Autodesk Fusion 360 part; units mm, degrees
note: some values were not read from the file. Set by a fixed rule: which sketch regions a step uses.
(part 3 of 3)
sketch "Sketch6" plane through (0, 0, 1) normal (0, 0, 1) x (-1, 0, 0)
  line L0 (-21.6697, -74.1094) -> (-35.669, -74.1094)
  line L1 (-35.669, -74.1094) -> (-35.669, -73.5101)
  line L2 (-35.669, -73.5101) -> (-36.4698, -73.5101)
  line L3 (-36.4698, -73.5101) -> (-36.4698, -60.7109)
  line L4 (-36.4698, -60.7109) -> (-35.669, -60.7109)
  line L5 (-35.669, -60.7109) -> (-35.669, -60.1102)
  line L6 (-35.669, -60.1102) -> (-21.6697, -60.1102)
  line L7 (-21.6697, -60.1102) -> (-21.6697, -60.7109)
  line L8 (-21.6697, -60.7109) -> (-20.869, -60.7109)
  line L9 (-20.869, -60.7109) -> (-20.869, -73.5101)
  line L10 (-20.869, -73.5101) -> (-21.6697, -73.5101)
  line L11 (-21.6697, -73.5101) -> (-21.6697, -74.1094)
  line L12 (-66.27, -35.585) -> (-69.07, -35.585)
  line L13 (-69.07, -35.585) -> (-69.07, -34.7597)
  line L14 (-69.07, -34.7597) -> (-72.3, -34.7597)
  line L15 (-72.3, -34.7597) -> (-72.3, -28.01)
  line L16 (-72.3, -28.01) -> (-69.07, -28.01)
  line L17 (-69.07, -28.01) -> (-69.07, -27.2852)
  line L18 (-69.07, -27.2852) -> (-73.1696, -27.2852)
  line L19 (-73.1696, -27.2852) -> (-73.1696, -26.4845)
  line L20 (-73.1696, -26.4845) -> (-73.769, -26.4845)
  line L21 (-73.769, -26.4845) -> (-73.769, -12.485)
  line L22 (-73.769, -12.485) -> (-73.1696, -12.485)
  line L23 (-73.1696, -12.485) -> (-73.1696, -11.6858)
  line L24 (-73.1696, -11.6858) -> (-69.07, -11.6858)
  line L25 (-69.07, -11.6858) -> (-69.07, -10.9595)
  line L26 (-69.07, -10.9595) -> (-72.3, -10.9595)
  line L27 (-72.3, -10.9595) -> (-72.3, -4.2099)
  line L28 (-72.3, -4.2099) -> (-69.07, -4.2099)
  line L29 (-69.07, -4.2099) -> (-69.07, -3.3858)
  line L30 (-69.07, -3.3858) -> (-66.27, -3.3858)
  line L31 (-66.27, -3.3858) -> (-66.27, -4.2099)
  line L32 (-66.27, -4.2099) -> (-59.9997, -4.2099)
  line L33 (-59.9997, -4.2099) -> (-59.9997, -5.9352)
  line L34 (-59.9997, -5.9352) -> (-58.7996, -5.9352)
  line L35 (-58.7996, -5.9352) -> (-58.7996, -9.2356)
  line L36 (-58.7996, -9.2356) -> (-59.9997, -9.2356)
  line L37 (-59.9997, -9.2356) -> (-59.9997, -10.9595)
  line L38 (-59.9997, -10.9595) -> (-64.4701, -10.9595)
  line L39 (-64.4701, -10.9595) -> (-64.4701, -11.6858)
  line L40 (-64.4701, -11.6858) -> (-60.3691, -11.6858)
  line L41 (-60.3691, -11.6858) -> (-60.3691, -12.485)
  line L42 (-60.3691, -12.485) -> (-59.7697, -12.485)
  line L43 (-59.7697, -12.485) -> (-59.7697, -26.4845)
  line L44 (-59.7697, -26.4845) -> (-60.3691, -26.4845)
  line L45 (-60.3691, -26.4845) -> (-60.3691, -27.2852)
  line L46 (-60.3691, -27.2852) -> (-64.4701, -27.2852)
  line L47 (-64.4701, -27.2852) -> (-64.4701, -28.01)
  line L48 (-64.4701, -28.01) -> (-59.9997, -28.01)
  line L49 (-59.9997, -28.01) -> (-59.9997, -29.7353)
  line L50 (-59.9997, -29.7353) -> (-58.7996, -29.7353)
  line L51 (-58.7996, -29.7353) -> (-58.7996, -33.0357)
  line L52 (-58.7996, -33.0357) -> (-59.9997, -33.0357)
  line L53 (-59.9997, -33.0357) -> (-59.9997, -34.7597)
  line L54 (-59.9997, -34.7597) -> (-66.27, -34.7597)
  line L55 (-66.27, -34.7597) -> (-66.27, -35.585)
  line L56 (-21.6697, -93.1594) -> (-35.669, -93.1594)
  line L57 (-35.669, -93.1594) -> (-35.669, -92.5601)
  line L58 (-35.669, -92.5601) -> (-36.4698, -92.5601)
  line L59 (-36.4698, -92.5601) -> (-36.4698, -79.7609)
  line L60 (-36.4698, -79.7609) -> (-35.669, -79.7609)
  line L61 (-35.669, -79.7609) -> (-35.669, -79.1602)
  line L62 (-35.669, -79.1602) -> (-21.6697, -79.1602)
  line L63 (-21.6697, -79.1602) -> (-21.6697, -79.7609)
  line L64 (-21.6697, -79.7609) -> (-20.869, -79.7609)
  line L65 (-20.869, -79.7609) -> (-20.869, -92.5601)
  line L66 (-20.869, -92.5601) -> (-21.6697, -92.5601)
  line L67 (-21.6697, -92.5601) -> (-21.6697, -93.1594)
  line L68 (-59.7697, -131.259) -> (-73.769, -131.259)
  line L69 (-73.769, -131.259) -> (-73.769, -130.66)
  line L70 (-73.769, -130.66) -> (-74.5698, -130.66)
  line L71 (-74.5698, -130.66) -> (-74.5698, -117.861)
  line L72 (-74.5698, -117.861) -> (-73.769, -117.861)
  line L73 (-73.769, -117.861) -> (-73.769, -117.26)
  line L74 (-73.769, -117.26) -> (-59.7697, -117.26)
  line L75 (-59.7697, -117.26) -> (-59.7697, -117.861)
  line L76 (-59.7697, -117.861) -> (-58.9689, -117.861)
  line L77 (-58.9689, -117.861) -> (-58.9689, -130.66)
  line L78 (-58.9689, -130.66) -> (-59.7697, -130.66)
  line L79 (-59.7697, -130.66) -> (-59.7697, -131.259)
  line L80 (-66.27, -73.685) -> (-69.07, -73.685)
  line L81 (-69.07, -73.685) -> (-69.07, -72.8595)
  line L82 (-69.07, -72.8595) -> (-72.3, -72.8595)
  line L83 (-72.3, -72.8595) -> (-72.3, -66.1098)
  line L84 (-72.3, -66.1098) -> (-69.07, -66.1098)
  line L85 (-69.07, -66.1098) -> (-69.07, -65.3852)
  line L86 (-69.07, -65.3852) -> (-73.1696, -65.3852)
  line L87 (-73.1696, -65.3852) -> (-73.1696, -64.5844)
  line L88 (-73.1696, -64.5844) -> (-73.769, -64.5844)
  line L89 (-73.769, -64.5844) -> (-73.769, -50.5852)
  line L90 (-73.769, -50.5852) -> (-73.1696, -50.5852)
  line L91 (-73.1696, -50.5852) -> (-73.1696, -49.7858)
  line L92 (-73.1696, -49.7858) -> (-69.07, -49.7858)
  line L93 (-69.07, -49.7858) -> (-69.07, -49.0594)
  line L94 (-69.07, -49.0594) -> (-72.3, -49.0594)
  line L95 (-72.3, -49.0594) -> (-72.3, -42.31)
  line L96 (-72.3, -42.31) -> (-69.07, -42.31)
  line L97 (-69.07, -42.31) -> (-69.07, -41.486)
  line L98 (-69.07, -41.486) -> (-66.27, -41.486)
  line L99 (-66.27, -41.486) -> (-66.27, -42.31)
  line L100 (-66.27, -42.31) -> (-59.9997, -42.31)
  line L101 (-59.9997, -42.31) -> (-59.9997, -44.0351)
  line L102 (-59.9997, -44.0351) -> (-58.7996, -44.0351)
  line L103 (-58.7996, -44.0351) -> (-58.7996, -47.3357)
  line L104 (-58.7996, -47.3357) -> (-59.9997, -47.3357)
  line L105 (-59.9997, -47.3357) -> (-59.9997, -49.0594)
  line L106 (-59.9997, -49.0594) -> (-64.4701, -49.0594)
  line L107 (-64.4701, -49.0594) -> (-64.4701, -49.7858)
  line L108 (-64.4701, -49.7858) -> (-60.3691, -49.7858)
  line L109 (-60.3691, -49.7858) -> (-60.3691, -50.5852)
  line L110 (-60.3691, -50.5852) -> (-59.7697, -50.5852)
  line L111 (-59.7697, -50.5852) -> (-59.7697, -64.5844)
  line L112 (-59.7697, -64.5844) -> (-60.3691, -64.5844)
  line L113 (-60.3691, -64.5844) -> (-60.3691, -65.3852)
  line L114 (-60.3691, -65.3852) -> (-64.4701, -65.3852)
  line L115 (-64.4701, -65.3852) -> (-64.4701, -66.1098)
  line L116 (-64.4701, -66.1098) -> (-59.9997, -66.1098)
  line L117 (-59.9997, -66.1098) -> (-59.9997, -67.8353)
  line L118 (-59.9997, -67.8353) -> (-58.7996, -67.8353)
  line L119 (-58.7996, -67.8353) -> (-58.7996, -71.1359)
  line L120 (-58.7996, -71.1359) -> (-59.9997, -71.1359)
  line L121 (-59.9997, -71.1359) -> (-59.9997, -72.8595)
  line L122 (-59.9997, -72.8595) -> (-66.27, -72.8595)
  line L123 (-66.27, -72.8595) -> (-66.27, -73.685)
  line L124 (-2.6197, -74.1094) -> (-16.6192, -74.1094)
  line L125 (-16.6192, -74.1094) -> (-16.6192, -73.5101)
  line L126 (-16.6192, -73.5101) -> (-17.4198, -73.5101)
  line L127 (-17.4198, -73.5101) -> (-17.4198, -60.7109)
  line L128 (-17.4198, -60.7109) -> (-16.6192, -60.7109)
  line L129 (-16.6192, -60.7109) -> (-16.6192, -60.1102)
  line L130 (-16.6192, -60.1102) -> (-2.6196, -60.1102)
  line L131 (-2.6197, -60.1102) -> (-2.6197, -60.7109)
  line L132 (-2.6197, -60.7109) -> (-1.819, -60.7109)
  line L133 (-1.819, -60.7109) -> (-1.819, -73.5101)
  line L134 (-1.819, -73.5101) -> (-2.6197, -73.5101)
  line L135 (-2.6197, -73.5101) -> (-2.6197, -74.1094)
  line L136 (-59.7697, -93.1594) -> (-73.769, -93.1594)
  line L137 (-73.769, -93.1594) -> (-73.769, -92.5601)
  line L138 (-73.769, -92.5601) -> (-74.5698, -92.5601)
  line L139 (-74.5698, -92.5601) -> (-74.5698, -79.7609)
  line L140 (-74.5698, -79.7609) -> (-73.769, -79.7609)
  line L141 (-73.769, -79.7609) -> (-73.769, -79.1602)
  line L142 (-73.769, -79.1602) -> (-59.7697, -79.1602)
  line L143 (-59.7697, -79.1602) -> (-59.7697, -79.7609)
  line L144 (-59.7697, -79.7609) -> (-58.9689, -79.7609)
  line L145 (-58.9689, -79.7609) -> (-58.9689, -92.5601)
  line L146 (-58.9689, -92.5601) -> (-59.7697, -92.5601)
  line L147 (-59.7697, -92.5601) -> (-59.7697, -93.1594)
  line L148 (-40.7197, -93.1594) -> (-54.719, -93.1594)
  line L149 (-54.719, -93.1594) -> (-54.719, -92.5601)
  line L150 (-54.719, -92.5601) -> (-55.5198, -92.5601)
  line L151 (-55.5198, -92.5601) -> (-55.5198, -79.7609)
  line L152 (-55.5198, -79.7609) -> (-54.719, -79.7609)
  line L153 (-54.719, -79.7609) -> (-54.719, -79.1602)
  line L154 (-54.719, -79.1602) -> (-40.7197, -79.1602)
  line L155 (-40.7197, -79.1602) -> (-40.7197, -79.7609)
  line L156 (-40.7197, -79.7609) -> (-39.9189, -79.7609)
  line L157 (-39.9189, -79.7609) -> (-39.9189, -92.5601)
  line L158 (-39.9189, -92.5601) -> (-40.7197, -92.5601)
  line L159 (-40.7197, -92.5601) -> (-40.7197, -93.1594)
  line L160 (-2.6197, -36.0094) -> (-16.6192, -36.0094)
  line L161 (-16.6192, -36.0094) -> (-16.6192, -35.4101)
  line L162 (-16.6192, -35.4101) -> (-17.4198, -35.4101)
  line L163 (-17.4198, -35.4101) -> (-17.4198, -22.6109)
  line L164 (-17.4198, -22.6109) -> (-16.6192, -22.6109)
  line L165 (-16.6192, -22.6109) -> (-16.6192, -22.01)
  line L166 (-16.6192, -22.01) -> (-2.6196, -22.01)
  line L167 (-2.6197, -22.01) -> (-2.6197, -22.6109)
  line L168 (-2.6197, -22.6109) -> (-1.819, -22.6109)
  line L169 (-1.819, -22.6109) -> (-1.819, -35.4101)
  line L170 (-1.819, -35.4101) -> (-2.6197, -35.4101)
  line L171 (-2.6197, -35.4101) -> (-2.6197, -36.0094)
  line L172 (-2.6197, -55.0594) -> (-16.6192, -55.0594)
  line L173 (-16.6192, -55.0594) -> (-16.6192, -54.4601)
  line L174 (-16.6192, -54.4601) -> (-17.4198, -54.4601)
  line L175 (-17.4198, -54.4601) -> (-17.4198, -41.6609)
  line L176 (-17.4198, -41.6609) -> (-16.6192, -41.6609)
  line L177 (-16.6192, -41.6609) -> (-16.6192, -41.0602)
  line L178 (-16.6192, -41.0602) -> (-2.6196, -41.0602)
  line L179 (-2.6197, -41.0602) -> (-2.6197, -41.6609)
  line L180 (-2.6197, -41.6609) -> (-1.819, -41.6609)
  line L181 (-1.819, -41.6609) -> (-1.819, -54.4601)
  line L182 (-1.819, -54.4601) -> (-2.6197, -54.4601)
  line L183 (-2.6197, -54.4601) -> (-2.6197, -55.0594)
  line L184 (-21.6697, -55.0594) -> (-35.669, -55.0594)
  line L185 (-35.669, -55.0594) -> (-35.669, -54.4601)
  line L186 (-35.669, -54.4601) -> (-36.4698, -54.4601)
  line L187 (-36.4698, -54.4601) -> (-36.4698, -41.6609)
  line L188 (-36.4698, -41.6609) -> (-35.669, -41.6609)
  line L189 (-35.669, -41.6609) -> (-35.669, -41.0602)
  line L190 (-35.669, -41.0602) -> (-21.6697, -41.0602)
  line L191 (-21.6697, -41.0602) -> (-21.6697, -41.6609)
  line L192 (-21.6697, -41.6609) -> (-20.869, -41.6609)
  line L193 (-20.869, -41.6609) -> (-20.869, -54.4601)
  line L194 (-20.869, -54.4601) -> (-21.6697, -54.4601)
  line L195 (-21.6697, -54.4601) -> (-21.6697, -55.0594)
  line L196 (-40.7197, -74.1094) -> (-54.719, -74.1094)
  line L197 (-54.719, -74.1094) -> (-54.719, -73.5101)
  line L198 (-54.719, -73.5101) -> (-55.5198, -73.5101)
  line L199 (-55.5198, -73.5101) -> (-55.5198, -60.7109)
  line L200 (-55.5198, -60.7109) -> (-54.719, -60.7109)
  line L201 (-54.719, -60.7109) -> (-54.719, -60.1102)
  line L202 (-54.719, -60.1102) -> (-40.7197, -60.1102)
  line L203 (-40.7197, -60.1102) -> (-40.7197, -60.7109)
  line L204 (-40.7197, -60.7109) -> (-39.9189, -60.7109)
  line L205 (-39.9189, -60.7109) -> (-39.9189, -73.5101)
  line L206 (-39.9189, -73.5101) -> (-40.7197, -73.5101)
  line L207 (-40.7197, -73.5101) -> (-40.7197, -74.1094)
  line L208 (-12.1447, -16.9595) -> (-26.1441, -16.9595)
  line L209 (-26.1441, -16.9595) -> (-26.1441, -16.3601)
  line L210 (-26.1441, -16.3601) -> (-26.9448, -16.3601)
  line L211 (-26.9448, -16.3601) -> (-26.9448, -12.2604)
  line L212 (-26.9448, -12.2604) -> (-27.6696, -12.2604)
  line L213 (-27.6696, -12.2604) -> (-27.6696, -15.4905)
  line L214 (-27.6696, -15.4905) -> (-34.4193, -15.4905)
  line L215 (-34.4193, -15.4905) -> (-34.4193, -12.2604)
  line L216 (-34.4193, -12.2604) -> (-35.2447, -12.2604)
  line L217 (-35.2447, -12.2604) -> (-35.2447, -9.4602)
  line L218 (-35.2447, -9.4602) -> (-34.4193, -9.4602)
  line L219 (-34.4193, -9.4602) -> (-34.4193, -3.1902)
  line L220 (-34.4193, -3.1902) -> (-32.694, -3.1902)
  line L221 (-32.694, -3.1902) -> (-32.694, -1.9899)
  line L222 (-32.694, -1.9899) -> (-29.3949, -1.9899)
  line L223 (-29.3949, -1.9899) -> (-29.3949, -3.1902)
  line L224 (-29.3949, -3.1902) -> (-27.6696, -3.1902)
  line L225 (-27.6696, -3.1902) -> (-27.6696, -7.6605)
  line L226 (-27.6696, -7.6605) -> (-26.9448, -7.6605)
  line L227 (-26.9448, -7.6605) -> (-26.9448, -3.5609)
  line L228 (-26.9448, -3.5609) -> (-26.1441, -3.5609)
  line L229 (-26.1441, -3.5609) -> (-26.1441, -2.96)
  line L230 (-26.1441, -2.96) -> (-12.1447, -2.96)
  line L231 (-12.1447, -2.96) -> (-12.1447, -3.5609)
  line L232 (-12.1447, -3.5609) -> (-11.344, -3.5609)
  line L233 (-11.344, -3.5609) -> (-11.344, -7.6605)
  line L234 (-11.344, -7.6605) -> (-10.6192, -7.6605)
  line L235 (-10.6192, -7.6605) -> (-10.6192, -3.1902)
  line L236 (-10.6192, -3.1902) -> (-8.8939, -3.1902)
  line L237 (-8.8939, -3.1902) -> (-8.8939, -1.9899)
  line L238 (-8.8939, -1.9899) -> (-5.5948, -1.9899)
  line L239 (-5.5948, -1.9899) -> (-5.5948, -3.1902)
  line L240 (-5.5948, -3.1902) -> (-3.8695, -3.1902)
  line L241 (-3.8695, -3.1902) -> (-3.8695, -9.4602)
  line L242 (-3.8695, -9.4602) -> (-3.0441, -9.4602)
  line L243 (-3.0441, -9.4602) -> (-3.0441, -12.2604)
  line L244 (-3.0441, -12.2604) -> (-3.8695, -12.2604)
  line L245 (-3.8695, -12.2604) -> (-3.8695, -15.4905)
  line L246 (-3.8695, -15.4905) -> (-10.6192, -15.4905)
  line L247 (-10.6192, -15.4905) -> (-10.6192, -12.2604)
  line L248 (-10.6192, -12.2604) -> (-11.344, -12.2604)
  line L249 (-11.344, -12.2604) -> (-11.344, -16.3601)
  line L250 (-11.344, -16.3601) -> (-12.1447, -16.3601)
  line L251 (-12.1447, -16.3601) -> (-12.1447, -16.9595)
  line L252 (-40.7197, -36.0094) -> (-54.719, -36.0094)
  line L253 (-54.719, -36.0094) -> (-54.719, -35.4101)
  line L254 (-54.719, -35.4101) -> (-55.5198, -35.4101)
  line L255 (-55.5198, -35.4101) -> (-55.5198, -22.6109)
  line L256 (-55.5198, -22.6109) -> (-54.719, -22.6109)
  line L257 (-54.719, -22.6109) -> (-54.719, -22.01)
  line L258 (-54.719, -22.01) -> (-40.7197, -22.01)
  line L259 (-40.7197, -22.01) -> (-40.7197, -22.6109)
  line L260 (-40.7197, -22.6109) -> (-39.9189, -22.6109)
  line L261 (-39.9189, -22.6109) -> (-39.9189, -35.4101)
  line L262 (-39.9189, -35.4101) -> (-40.7197, -35.4101)
  line L263 (-40.7197, -35.4101) -> (-40.7197, -36.0094)
  line L264 (-40.7197, -55.0594) -> (-54.719, -55.0594)
  line L265 (-54.719, -55.0594) -> (-54.719, -54.4601)
  line L266 (-54.719, -54.4601) -> (-55.5198, -54.4601)
  line L267 (-55.5198, -54.4601) -> (-55.5198, -41.6609)
  line L268 (-55.5198, -41.6609) -> (-54.719, -41.6609)
  line L269 (-54.719, -41.6609) -> (-54.719, -41.0602)
  line L270 (-54.719, -41.0602) -> (-40.7197, -41.0602)
  line L271 (-40.7197, -41.0602) -> (-40.7197, -41.6609)
  line L272 (-40.7197, -41.6609) -> (-39.9189, -41.6609)
  line L273 (-39.9189, -41.6609) -> (-39.9189, -54.4601)
  line L274 (-39.9189, -54.4601) -> (-40.7197, -54.4601)
  line L275 (-40.7197, -54.4601) -> (-40.7197, -55.0594)
  line L276 (-21.6697, -36.0094) -> (-35.669, -36.0094)
  line L277 (-35.669, -36.0094) -> (-35.669, -35.4101)
  line L278 (-35.669, -35.4101) -> (-36.4698, -35.4101)
  line L279 (-36.4698, -35.4101) -> (-36.4698, -22.6109)
  line L280 (-36.4698, -22.6109) -> (-35.669, -22.6109)
  line L281 (-35.669, -22.6109) -> (-35.669, -22.01)
  line L282 (-35.669, -22.01) -> (-21.6697, -22.01)
  line L283 (-21.6697, -22.01) -> (-21.6697, -22.6109)
  line L284 (-21.6697, -22.6109) -> (-20.869, -22.6109)
  line L285 (-20.869, -22.6109) -> (-20.869, -35.4101)
  line L286 (-20.869, -35.4101) -> (-21.6697, -35.4101)
  line L287 (-21.6697, -35.4101) -> (-21.6697, -36.0094)
  line L288 (-2.6197, -93.1594) -> (-16.6192, -93.1594)
  line L289 (-16.6192, -93.1594) -> (-16.6192, -92.5601)
  line L290 (-16.6192, -92.5601) -> (-17.4198, -92.5601)
  line L291 (-17.4198, -92.5601) -> (-17.4198, -79.7609)
  line L292 (-17.4198, -79.7609) -> (-16.6192, -79.7609)
  line L293 (-16.6192, -79.7609) -> (-16.6192, -79.1602)
  line L294 (-16.6192, -79.1602) -> (-2.6196, -79.1602)
  line L295 (-2.6197, -79.1602) -> (-2.6197, -79.7609)
  line L296 (-2.6197, -79.7609) -> (-1.819, -79.7609)
  line L297 (-1.819, -79.7609) -> (-1.819, -92.5601)
  line L298 (-1.819, -92.5601) -> (-2.6197, -92.5601)
  line L299 (-2.6197, -92.5601) -> (-2.6197, -93.1594)
  line L300 (-40.7197, -16.9595) -> (-54.719, -16.9595)
  line L301 (-54.719, -16.9595) -> (-54.719, -16.3601)
  line L302 (-54.719, -16.3601) -> (-55.5198, -16.3601)
  line L303 (-55.5198, -16.3601) -> (-55.5198, -3.5609)
  line L304 (-55.5198, -3.5609) -> (-54.719, -3.5609)
  line L305 (-54.719, -3.5609) -> (-54.719, -2.96)
  line L306 (-54.719, -2.96) -> (-40.7197, -2.96)
  line L307 (-40.7197, -2.96) -> (-40.7197, -3.5609)
  line L308 (-40.7197, -3.5609) -> (-39.9189, -3.5609)
  line L309 (-39.9189, -3.5609) -> (-39.9189, -16.3601)
  line L310 (-39.9189, -16.3601) -> (-40.7197, -16.3601)
  line L311 (-40.7197, -16.3601) -> (-40.7197, -16.9595)
  line L312 (-87.4343, -163.6) -> (11.1659, -163.6)
  line L313 (11.1659, -163.6) -> (11.1659, 14.2999)
  line L314 (11.1659, 14.2999) -> (-87.4343, 14.2999)
  line L315 (-87.4343, 14.2999) -> (-87.4343, -163.6)
  line L316 (11.1659, -163.6) -> (-82.4343, -163.6)
  line L317 (-82.4343, -163.6) -> (-82.4343, 14.2999)
  line L318 (-82.4343, 14.2999) -> (11.1659, 14.2999)
  line L319 (11.1659, 14.2999) -> (11.1659, -163.6)
  line L320 (6.1659, -163.6) -> (6.1659, 48.0754)
  line L321 (30.3811, 8.3643) -> (-115.8718, 8.3643)
  line L322 (-117.8089, -158.6) -> (57.0165, -158.6)
  dimension "d59" = 5
  dimension "d60" = 5
  dimension "d61" = 5
  dimension "d62" = 5.9356
  constraint horizontal L316
  constraint vertical L317
  constraint horizontal L318
  constraint vertical L319
  constraint coincident L314 L317.end
  constraint coincident L312.end L313.start
  constraint coincident L312 L320.start
  constraint perpendicular L318 L320
  constraint perpendicular L313 L321
  constraint horizontal L322
  measures "d59" distance of L315 L317
  measures "d60" distance of L316 L322
  measures "d61" distance of L319 L320
  measures "d62" distance of L318 L321
extrude "Extrude22" add sketch "Sketch5" along normal blind 15 separate body contours L316 L317 L318 L319 L320 L321 L322 L323 makes body 4
combine "Combine1" operation add target body 3 tool bodies 4
sketch "Sketch7" plane through (0, 0, 19) normal (0, 0, 1) x (-1, 0, 0)
  line L0 (-87.4343, -163.6) -> (-87.4343, 14.2999)
  line L1 (-87.4343, 14.2999) -> (11.1659, 14.2999)
  line L2 (11.1659, 14.2999) -> (11.1659, -163.6)
  line L3 (11.1659, -163.6) -> (-87.4343, -163.6)
  line L4 (-92.4343, 19.2999) -> (-92.4343, -168.6)
  line L5 (-92.4343, -168.6) -> (16.1659, -168.6)
  line L6 (16.1659, -168.6) -> (16.1659, 19.2999)
  line L7 (16.1659, 19.2999) -> (-92.4343, 19.2999)
  line L8 (6.1659, -158.6) -> (6.1659, 9.2999)
  line L9 (-82.4343, -158.6) -> (-82.4343, 9.2999)
  line L10 (-82.4343, -158.6) -> (6.1659, -158.6)
  line L11 (6.1659, 9.2999) -> (-82.4343, 9.2999)
extrude "Extrude23" add sketch "Sketch7" against normal blind 15 from surface at -3 contours L0 L1 L2 L3 bodies 3
sketch "Sketch8" plane through (92.4343, 0, 0) normal (1, 0, 0) x (0, 1, 0)
  line L0 (168.6, 1) -> (168.6, 19)
  line L1 (168.6, 19) -> (-19.2999, 19)
  line L2 (-19.2999, 19) -> (-19.2999, 1)
  line L3 (-19.2999, 1) -> (168.6, 1)
  line L4 (168.6, 1) -> (168.6, -14)
  line L5 (168.6, -14) -> (-19.2999, 1)
  dimension "d72" = 15
  constraint coincident L0.start L3.end
  constraint perpendicular L3 L4
  constraint coincident L2.end L3.start
  measures "d72" distance of L0.start L4.end
extrude "Extrude24" add sketch "Sketch8" against normal blind 108.6 contours L3 L4 L5 bodies 3
move_body "Move1" bodies 1 to x (1, 0, 0) y (0, 1, 0) z (0, 0, 1) at (0, 0, 18)
sketch "Sketch9" plane through (0, 0, 19) normal (0, 0, 1) x (-1, 0, 0)
  line L0 (-21.6697, -74.1094) -> (-35.669, -74.1094)
  line L1 (-35.669, -74.1094) -> (-35.669, -73.5101)
  line L2 (-35.669, -73.5101) -> (-36.4698, -73.5101)
  line L3 (-36.4698, -73.5101) -> (-36.4698, -60.7109)
  line L4 (-36.4698, -60.7109) -> (-35.669, -60.7109)
  line L5 (-35.669, -60.7109) -> (-35.669, -60.1102)
  line L6 (-35.669, -60.1102) -> (-21.6697, -60.1102)
  line L7 (-21.6697, -60.1102) -> (-21.6697, -60.7109)
  line L8 (-21.6697, -60.7109) -> (-20.869, -60.7109)
  line L9 (-20.869, -60.7109) -> (-20.869, -73.5101)
  line L10 (-20.869, -73.5101) -> (-21.6697, -73.5101)
  line L11 (-21.6697, -73.5101) -> (-21.6697, -74.1094)
  line L12 (-66.27, -35.585) -> (-69.07, -35.585)
  line L13 (-69.07, -35.585) -> (-69.07, -34.7597)
  line L14 (-69.07, -34.7597) -> (-72.3, -34.7597)
  line L15 (-72.3, -34.7597) -> (-72.3, -28.01)
  line L16 (-72.3, -28.01) -> (-69.07, -28.01)
  line L17 (-69.07, -28.01) -> (-69.07, -27.2852)
  line L18 (-69.07, -27.2852) -> (-73.1696, -27.2852)
  line L19 (-73.1696, -27.2852) -> (-73.1696, -26.4845)
  line L20 (-73.1696, -26.4845) -> (-73.769, -26.4845)
  line L21 (-73.769, -26.4845) -> (-73.769, -12.485)
  line L22 (-73.769, -12.485) -> (-73.1696, -12.485)
  line L23 (-73.1696, -12.485) -> (-73.1696, -11.6858)
  line L24 (-73.1696, -11.6858) -> (-69.07, -11.6858)
  line L25 (-69.07, -11.6858) -> (-69.07, -10.9595)
  line L26 (-69.07, -10.9595) -> (-72.3, -10.9595)
  line L27 (-72.3, -10.9595) -> (-72.3, -4.2099)
  line L28 (-72.3, -4.2099) -> (-69.07, -4.2099)
  line L29 (-69.07, -4.2099) -> (-69.07, -3.3858)
  line L30 (-69.07, -3.3858) -> (-66.27, -3.3858)
  line L31 (-66.27, -3.3858) -> (-66.27, -4.2099)
  line L32 (-66.27, -4.2099) -> (-59.9997, -4.2099)
  line L33 (-59.9997, -4.2099) -> (-59.9997, -5.9352)
  line L34 (-59.9997, -5.9352) -> (-58.7996, -5.9352)
  line L35 (-58.7996, -5.9352) -> (-58.7996, -9.2356)
  line L36 (-58.7996, -9.2356) -> (-59.9997, -9.2356)
  line L37 (-59.9997, -9.2356) -> (-59.9997, -10.9595)
  line L38 (-59.9997, -10.9595) -> (-64.4701, -10.9595)
  line L39 (-64.4701, -10.9595) -> (-64.4701, -11.6858)
  line L40 (-64.4701, -11.6858) -> (-60.3691, -11.6858)
  line L41 (-60.3691, -11.6858) -> (-60.3691, -12.485)
  line L42 (-60.3691, -12.485) -> (-59.7697, -12.485)
  line L43 (-59.7697, -12.485) -> (-59.7697, -26.4845)
  line L44 (-59.7697, -26.4845) -> (-60.3691, -26.4845)
  line L45 (-60.3691, -26.4845) -> (-60.3691, -27.2852)
  line L46 (-60.3691, -27.2852) -> (-64.4701, -27.2852)
  line L47 (-64.4701, -27.2852) -> (-64.4701, -28.01)
  line L48 (-64.4701, -28.01) -> (-59.9997, -28.01)
  line L49 (-59.9997, -28.01) -> (-59.9997, -29.7353)
  line L50 (-59.9997, -29.7353) -> (-58.7996, -29.7353)
  line L51 (-58.7996, -29.7353) -> (-58.7996, -33.0357)
  line L52 (-58.7996, -33.0357) -> (-59.9997, -33.0357)
  line L53 (-59.9997, -33.0357) -> (-59.9997, -34.7597)
  line L54 (-59.9997, -34.7597) -> (-66.27, -34.7597)
  line L55 (-66.27, -34.7597) -> (-66.27, -35.585)
  line L56 (-21.6697, -93.1594) -> (-35.669, -93.1594)
  line L57 (-35.669, -93.1594) -> (-35.669, -92.5601)
  line L58 (-35.669, -92.5601) -> (-36.4698, -92.5601)
  line L59 (-36.4698, -92.5601) -> (-36.4698, -79.7609)
  line L60 (-36.4698, -79.7609) -> (-35.669, -79.7609)
  line L61 (-35.669, -79.7609) -> (-35.669, -79.1602)
  line L62 (-35.669, -79.1602) -> (-21.6697, -79.1602)
  line L63 (-21.6697, -79.1602) -> (-21.6697, -79.7609)
  line L64 (-21.6697, -79.7609) -> (-20.869, -79.7609)
  line L65 (-20.869, -79.7609) -> (-20.869, -92.5601)
  line L66 (-20.869, -92.5601) -> (-21.6697, -92.5601)
  line L67 (-21.6697, -92.5601) -> (-21.6697, -93.1594)
  line L68 (-59.7697, -131.259) -> (-73.769, -131.259)
  line L69 (-73.769, -131.259) -> (-73.769, -130.66)
  line L70 (-73.769, -130.66) -> (-74.5698, -130.66)
  line L71 (-74.5698, -130.66) -> (-74.5698, -117.861)
  line L72 (-74.5698, -117.861) -> (-73.769, -117.861)
  line L73 (-73.769, -117.861) -> (-73.769, -117.26)
  line L74 (-73.769, -117.26) -> (-59.7697, -117.26)
  line L75 (-59.7697, -117.26) -> (-59.7697, -117.861)
  line L76 (-59.7697, -117.861) -> (-58.9689, -117.861)
  line L77 (-58.9689, -117.861) -> (-58.9689, -130.66)
  line L78 (-58.9689, -130.66) -> (-59.7697, -130.66)
  line L79 (-59.7697, -130.66) -> (-59.7697, -131.259)
  line L80 (-66.27, -73.685) -> (-69.07, -73.685)
  line L81 (-69.07, -73.685) -> (-69.07, -72.8595)
  line L82 (-69.07, -72.8595) -> (-72.3, -72.8595)
  line L83 (-72.3, -72.8595) -> (-72.3, -66.1098)
  line L84 (-72.3, -66.1098) -> (-69.07, -66.1098)
  line L85 (-69.07, -66.1098) -> (-69.07, -65.3852)
  line L86 (-69.07, -65.3852) -> (-73.1696, -65.3852)
  line L87 (-73.1696, -65.3852) -> (-73.1696, -64.5844)
  line L88 (-73.1696, -64.5844) -> (-73.769, -64.5844)
  line L89 (-73.769, -64.5844) -> (-73.769, -50.5852)
  line L90 (-73.769, -50.5852) -> (-73.1696, -50.5852)
  line L91 (-73.1696, -50.5852) -> (-73.1696, -49.7858)
  line L92 (-73.1696, -49.7858) -> (-69.07, -49.7858)
  line L93 (-69.07, -49.7858) -> (-69.07, -49.0594)
  line L94 (-69.07, -49.0594) -> (-72.3, -49.0594)
  line L95 (-72.3, -49.0594) -> (-72.3, -42.31)
  line L96 (-72.3, -42.31) -> (-69.07, -42.31)
  line L97 (-69.07, -42.31) -> (-69.07, -41.486)
  line L98 (-69.07, -41.486) -> (-66.27, -41.486)
  line L99 (-66.27, -41.486) -> (-66.27, -42.31)
  line L100 (-66.27, -42.31) -> (-59.9997, -42.31)
  line L101 (-59.9997, -42.31) -> (-59.9997, -44.0351)
  line L102 (-59.9997, -44.0351) -> (-58.7996, -44.0351)
  line L103 (-58.7996, -44.0351) -> (-58.7996, -47.3357)
  line L104 (-58.7996, -47.3357) -> (-59.9997, -47.3357)
  line L105 (-59.9997, -47.3357) -> (-59.9997, -49.0594)
  line L106 (-59.9997, -49.0594) -> (-64.4701, -49.0594)
  line L107 (-64.4701, -49.0594) -> (-64.4701, -49.7858)
  line L108 (-64.4701, -49.7858) -> (-60.3691, -49.7858)
  line L109 (-60.3691, -49.7858) -> (-60.3691, -50.5852)
  line L110 (-60.3691, -50.5852) -> (-59.7697, -50.5852)
  line L111 (-59.7697, -50.5852) -> (-59.7697, -64.5844)
  line L112 (-59.7697, -64.5844) -> (-60.3691, -64.5844)
  line L113 (-60.3691, -64.5844) -> (-60.3691, -65.3852)
  line L114 (-60.3691, -65.3852) -> (-64.4701, -65.3852)
  line L115 (-64.4701, -65.3852) -> (-64.4701, -66.1098)
  line L116 (-64.4701, -66.1098) -> (-59.9997, -66.1098)
  line L117 (-59.9997, -66.1098) -> (-59.9997, -67.8353)
  line L118 (-59.9997, -67.8353) -> (-58.7996, -67.8353)
  line L119 (-58.7996, -67.8353) -> (-58.7996, -71.1359)
  line L120 (-58.7996, -71.1359) -> (-59.9997, -71.1359)
  line L121 (-59.9997, -71.1359) -> (-59.9997, -72.8595)
  line L122 (-59.9997, -72.8595) -> (-66.27, -72.8595)
  line L123 (-66.27, -72.8595) -> (-66.27, -73.685)
  line L124 (-2.6197, -74.1094) -> (-16.6192, -74.1094)
  line L125 (-16.6192, -74.1094) -> (-16.6192, -73.5101)
  line L126 (-16.6192, -73.5101) -> (-17.4198, -73.5101)
  line L127 (-17.4198, -73.5101) -> (-17.4198, -60.7109)
  line L128 (-17.4198, -60.7109) -> (-16.6192, -60.7109)
  line L129 (-16.6192, -60.7109) -> (-16.6192, -60.1102)
  line L130 (-16.6192, -60.1102) -> (-2.6196, -60.1102)
  line L131 (-2.6197, -60.1102) -> (-2.6197, -60.7109)
  line L132 (-2.6197, -60.7109) -> (-1.819, -60.7109)
  line L133 (-1.819, -60.7109) -> (-1.819, -73.5101)
  line L134 (-1.819, -73.5101) -> (-2.6197, -73.5101)
  line L135 (-2.6197, -73.5101) -> (-2.6197, -74.1094)
  line L136 (-59.7697, -93.1594) -> (-73.769, -93.1594)
  line L137 (-73.769, -93.1594) -> (-73.769, -92.5601)
  line L138 (-73.769, -92.5601) -> (-74.5698, -92.5601)
  line L139 (-74.5698, -92.5601) -> (-74.5698, -79.7609)
  line L140 (-74.5698, -79.7609) -> (-73.769, -79.7609)
  line L141 (-73.769, -79.7609) -> (-73.769, -79.1602)
  line L142 (-73.769, -79.1602) -> (-59.7697, -79.1602)
  line L143 (-59.7697, -79.1602) -> (-59.7697, -79.7609)
  line L144 (-59.7697, -79.7609) -> (-58.9689, -79.7609)
  line L145 (-58.9689, -79.7609) -> (-58.9689, -92.5601)
  line L146 (-58.9689, -92.5601) -> (-59.7697, -92.5601)
  line L147 (-59.7697, -92.5601) -> (-59.7697, -93.1594)
  line L148 (-40.7197, -93.1594) -> (-54.719, -93.1594)
  line L149 (-54.719, -93.1594) -> (-54.719, -92.5601)
  line L150 (-54.719, -92.5601) -> (-55.5198, -92.5601)
  line L151 (-55.5198, -92.5601) -> (-55.5198, -79.7609)
  line L152 (-55.5198, -79.7609) -> (-54.719, -79.7609)
  line L153 (-54.719, -79.7609) -> (-54.719, -79.1602)
  line L154 (-54.719, -79.1602) -> (-40.7197, -79.1602)
  line L155 (-40.7197, -79.1602) -> (-40.7197, -79.7609)
  line L156 (-40.7197, -79.7609) -> (-39.9189, -79.7609)
  line L157 (-39.9189, -79.7609) -> (-39.9189, -92.5601)
  line L158 (-39.9189, -92.5601) -> (-40.7197, -92.5601)
  line L159 (-40.7197, -92.5601) -> (-40.7197, -93.1594)
  line L160 (-2.6197, -36.0094) -> (-16.6192, -36.0094)
  line L161 (-16.6192, -36.0094) -> (-16.6192, -35.4101)
  line L162 (-16.6192, -35.4101) -> (-17.4198, -35.4101)
  line L163 (-17.4198, -35.4101) -> (-17.4198, -22.6109)
  line L164 (-17.4198, -22.6109) -> (-16.6192, -22.6109)
  line L165 (-16.6192, -22.6109) -> (-16.6192, -22.01)
  line L166 (-16.6192, -22.01) -> (-2.6196, -22.01)
  line L167 (-2.6197, -22.01) -> (-2.6197, -22.6109)
  line L168 (-2.6197, -22.6109) -> (-1.819, -22.6109)
  line L169 (-1.819, -22.6109) -> (-1.819, -35.4101)
  line L170 (-1.819, -35.4101) -> (-2.6197, -35.4101)
  line L171 (-2.6197, -35.4101) -> (-2.6197, -36.0094)
  line L172 (-2.6197, -55.0594) -> (-16.6192, -55.0594)
  line L173 (-16.6192, -55.0594) -> (-16.6192, -54.4601)
  line L174 (-16.6192, -54.4601) -> (-17.4198, -54.4601)
  line L175 (-17.4198, -54.4601) -> (-17.4198, -41.6609)
  line L176 (-17.4198, -41.6609) -> (-16.6192, -41.6609)
  line L177 (-16.6192, -41.6609) -> (-16.6192, -41.0602)
  line L178 (-16.6192, -41.0602) -> (-2.6196, -41.0602)
  line L179 (-2.6197, -41.0602) -> (-2.6197, -41.6609)
  line L180 (-2.6197, -41.6609) -> (-1.819, -41.6609)
  line L181 (-1.819, -41.6609) -> (-1.819, -54.4601)
  line L182 (-1.819, -54.4601) -> (-2.6197, -54.4601)
  line L183 (-2.6197, -54.4601) -> (-2.6197, -55.0594)
  line L184 (-21.6697, -55.0594) -> (-35.669, -55.0594)
  line L185 (-35.669, -55.0594) -> (-35.669, -54.4601)
  line L186 (-35.669, -54.4601) -> (-36.4698, -54.4601)
  line L187 (-36.4698, -54.4601) -> (-36.4698, -41.6609)
  line L188 (-36.4698, -41.6609) -> (-35.669, -41.6609)
  line L189 (-35.669, -41.6609) -> (-35.669, -41.0602)
  line L190 (-35.669, -41.0602) -> (-21.6697, -41.0602)
  line L191 (-21.6697, -41.0602) -> (-21.6697, -41.6609)
  line L192 (-21.6697, -41.6609) -> (-20.869, -41.6609)
  line L193 (-20.869, -41.6609) -> (-20.869, -54.4601)
  line L194 (-20.869, -54.4601) -> (-21.6697, -54.4601)
  line L195 (-21.6697, -54.4601) -> (-21.6697, -55.0594)
  line L196 (-40.7197, -74.1094) -> (-54.719, -74.1094)
  line L197 (-54.719, -74.1094) -> (-54.719, -73.5101)
  line L198 (-54.719, -73.5101) -> (-55.5198, -73.5101)
  line L199 (-55.5198, -73.5101) -> (-55.5198, -60.7109)
  line L200 (-55.5198, -60.7109) -> (-54.719, -60.7109)
  line L201 (-54.719, -60.7109) -> (-54.719, -60.1102)
  line L202 (-54.719, -60.1102) -> (-40.7197, -60.1102)
  line L203 (-40.7197, -60.1102) -> (-40.7197, -60.7109)
  line L204 (-40.7197, -60.7109) -> (-39.9189, -60.7109)
  line L205 (-39.9189, -60.7109) -> (-39.9189, -73.5101)
  line L206 (-39.9189, -73.5101) -> (-40.7197, -73.5101)
  line L207 (-40.7197, -73.5101) -> (-40.7197, -74.1094)
  line L208 (-12.1447, -16.9595) -> (-26.1441, -16.9595)
  line L209 (-26.1441, -16.9595) -> (-26.1441, -16.3601)
  line L210 (-26.1441, -16.3601) -> (-26.9448, -16.3601)
  line L211 (-26.9448, -16.3601) -> (-26.9448, -12.2604)
  line L212 (-26.9448, -12.2604) -> (-27.6696, -12.2604)
  line L213 (-27.6696, -12.2604) -> (-27.6696, -15.4905)
  line L214 (-27.6696, -15.4905) -> (-34.4193, -15.4905)
  line L215 (-34.4193, -15.4905) -> (-34.4193, -12.2604)
  line L216 (-34.4193, -12.2604) -> (-35.2447, -12.2604)
  line L217 (-35.2447, -12.2604) -> (-35.2447, -9.4602)
  line L218 (-35.2447, -9.4602) -> (-34.4193, -9.4602)
  line L219 (-34.4193, -9.4602) -> (-34.4193, -3.1902)
  line L220 (-34.4193, -3.1902) -> (-32.694, -3.1902)
  line L221 (-32.694, -3.1902) -> (-32.694, -1.9899)
  line L222 (-32.694, -1.9899) -> (-29.3949, -1.9899)
  line L223 (-29.3949, -1.9899) -> (-29.3949, -3.1902)
  line L224 (-29.3949, -3.1902) -> (-27.6696, -3.1902)
  line L225 (-27.6696, -3.1902) -> (-27.6696, -7.6605)
  line L226 (-27.6696, -7.6605) -> (-26.9448, -7.6605)
  line L227 (-26.9448, -7.6605) -> (-26.9448, -3.5609)
  line L228 (-26.9448, -3.5609) -> (-26.1441, -3.5609)
  line L229 (-26.1441, -3.5609) -> (-26.1441, -2.96)
  line L230 (-26.1441, -2.96) -> (-12.1447, -2.96)
  line L231 (-12.1447, -2.96) -> (-12.1447, -3.5609)
  line L232 (-12.1447, -3.5609) -> (-11.344, -3.5609)
  line L233 (-11.344, -3.5609) -> (-11.344, -7.6605)
  line L234 (-11.344, -7.6605) -> (-10.6192, -7.6605)
  line L235 (-10.6192, -7.6605) -> (-10.6192, -3.1902)
  line L236 (-10.6192, -3.1902) -> (-8.8939, -3.1902)
  line L237 (-8.8939, -3.1902) -> (-8.8939, -1.9899)
  line L238 (-8.8939, -1.9899) -> (-5.5948, -1.9899)
  line L239 (-5.5948, -1.9899) -> (-5.5948, -3.1902)
  line L240 (-5.5948, -3.1902) -> (-3.8695, -3.1902)
  line L241 (-3.8695, -3.1902) -> (-3.8695, -9.4602)
  line L242 (-3.8695, -9.4602) -> (-3.0441, -9.4602)
  line L243 (-3.0441, -9.4602) -> (-3.0441, -12.2604)
  line L244 (-3.0441, -12.2604) -> (-3.8695, -12.2604)
  line L245 (-3.8695, -12.2604) -> (-3.8695, -15.4905)
  line L246 (-3.8695, -15.4905) -> (-10.6192, -15.4905)
  line L247 (-10.6192, -15.4905) -> (-10.6192, -12.2604)
  line L248 (-10.6192, -12.2604) -> (-11.344, -12.2604)
  line L249 (-11.344, -12.2604) -> (-11.344, -16.3601)
  line L250 (-11.344, -16.3601) -> (-12.1447, -16.3601)
  line L251 (-12.1447, -16.3601) -> (-12.1447, -16.9595)
  line L252 (-40.7197, -36.0094) -> (-54.719, -36.0094)
  line L253 (-54.719, -36.0094) -> (-54.719, -35.4101)
  line L254 (-54.719, -35.4101) -> (-55.5198, -35.4101)
  line L255 (-55.5198, -35.4101) -> (-55.5198, -22.6109)
  line L256 (-55.5198, -22.6109) -> (-54.719, -22.6109)
  line L257 (-54.719, -22.6109) -> (-54.719, -22.01)
  line L258 (-54.719, -22.01) -> (-40.7197, -22.01)
  line L259 (-40.7197, -22.01) -> (-40.7197, -22.6109)
  line L260 (-40.7197, -22.6109) -> (-39.9189, -22.6109)
  line L261 (-39.9189, -22.6109) -> (-39.9189, -35.4101)
  line L262 (-39.9189, -35.4101) -> (-40.7197, -35.4101)
  line L263 (-40.7197, -35.4101) -> (-40.7197, -36.0094)
  line L264 (-40.7197, -55.0594) -> (-54.719, -55.0594)
  line L265 (-54.719, -55.0594) -> (-54.719, -54.4601)
  line L266 (-54.719, -54.4601) -> (-55.5198, -54.4601)
  line L267 (-55.5198, -54.4601) -> (-55.5198, -41.6609)
  line L268 (-55.5198, -41.6609) -> (-54.719, -41.6609)
  line L269 (-54.719, -41.6609) -> (-54.719, -41.0602)
  line L270 (-54.719, -41.0602) -> (-40.7197, -41.0602)
  line L271 (-40.7197, -41.0602) -> (-40.7197, -41.6609)
  line L272 (-40.7197, -41.6609) -> (-39.9189, -41.6609)
  line L273 (-39.9189, -41.6609) -> (-39.9189, -54.4601)
  line L274 (-39.9189, -54.4601) -> (-40.7197, -54.4601)
  line L275 (-40.7197, -54.4601) -> (-40.7197, -55.0594)
  line L276 (-21.6697, -36.0094) -> (-35.669, -36.0094)
  line L277 (-35.669, -36.0094) -> (-35.669, -35.4101)
  line L278 (-35.669, -35.4101) -> (-36.4698, -35.4101)
  line L279 (-36.4698, -35.4101) -> (-36.4698, -22.6109)
  line L280 (-36.4698, -22.6109) -> (-35.669, -22.6109)
  line L281 (-35.669, -22.6109) -> (-35.669, -22.01)
  line L282 (-35.669, -22.01) -> (-21.6697, -22.01)
  line L283 (-21.6697, -22.01) -> (-21.6697, -22.6109)
  line L284 (-21.6697, -22.6109) -> (-20.869, -22.6109)
  line L285 (-20.869, -22.6109) -> (-20.869, -35.4101)
  line L286 (-20.869, -35.4101) -> (-21.6697, -35.4101)
  line L287 (-21.6697, -35.4101) -> (-21.6697, -36.0094)
  line L288 (-2.6197, -93.1594) -> (-16.6192, -93.1594)
  line L289 (-16.6192, -93.1594) -> (-16.6192, -92.5601)
  line L290 (-16.6192, -92.5601) -> (-17.4198, -92.5601)
  line L291 (-17.4198, -92.5601) -> (-17.4198, -79.7609)
  line L292 (-17.4198, -79.7609) -> (-16.6192, -79.7609)
  line L293 (-16.6192, -79.7609) -> (-16.6192, -79.1602)
  line L294 (-16.6192, -79.1602) -> (-2.6196, -79.1602)
  line L295 (-2.6197, -79.1602) -> (-2.6197, -79.7609)
  line L296 (-2.6197, -79.7609) -> (-1.819, -79.7609)
  line L297 (-1.819, -79.7609) -> (-1.819, -92.5601)
  line L298 (-1.819, -92.5601) -> (-2.6197, -92.5601)
  line L299 (-2.6197, -92.5601) -> (-2.6197, -93.1594)
  line L300 (-40.7197, -16.9595) -> (-54.719, -16.9595)
  line L301 (-54.719, -16.9595) -> (-54.719, -16.3601)
  line L302 (-54.719, -16.3601) -> (-55.5198, -16.3601)
  line L303 (-55.5198, -16.3601) -> (-55.5198, -3.5609)
  line L304 (-55.5198, -3.5609) -> (-54.719, -3.5609)
  line L305 (-54.719, -3.5609) -> (-54.719, -2.96)
  line L306 (-54.719, -2.96) -> (-40.7197, -2.96)
  line L307 (-40.7197, -2.96) -> (-40.7197, -3.5609)
  line L308 (-40.7197, -3.5609) -> (-39.9189, -3.5609)
  line L309 (-39.9189, -3.5609) -> (-39.9189, -16.3601)
  line L310 (-39.9189, -16.3601) -> (-40.7197, -16.3601)
  line L311 (-40.7197, -16.3601) -> (-40.7197, -16.9595)
  line L312 (-87.4343, -163.6) -> (11.1659, -163.6)
  line L313 (11.1659, -163.6) -> (11.1659, 14.2999)
  line L314 (11.1659, 14.2999) -> (-87.4343, 14.2999)
  line L315 (-87.4343, 14.2999) -> (-87.4343, -163.6)
  line L316 (-38.1342, -163.6) -> (-38.1342, -174.7774)
  line L317 (-38.1342, -174.7774) -> (-38.1342, -163.6)
  line L318 (-38.1342, -163.6) -> (-38.1342, 43.927)
  line L319 (11.1659, -74.65) -> (-130.7073, -74.65)
  line L320 (11.1659, -74.65) -> (62.2305, -74.65)
  circle A0 centre (8.3275, -160.9728) radius 1.1
  line L321 (5.9026, -160.984) -> (7.1247, -163.0784)
  line L322 (7.1247, -163.0784) -> (9.5496, -163.0672)
  line L323 (9.5496, -163.0672) -> (10.7523, -160.9617)
  line L324 (10.7523, -160.9617) -> (9.5302, -158.8673)
  line L325 (9.5302, -158.8673) -> (7.1054, -158.8784)
  line L326 (7.1054, -158.8784) -> (5.9026, -160.984)
  circle A1 centre (-84.5959, -160.9728) radius 1.1
  line L327 (-85.7986, -158.8673) -> (-83.3738, -158.8784)
  line L328 (-83.3738, -158.8784) -> (-82.171, -160.984)
  line L329 (-82.171, -160.984) -> (-83.3931, -163.0784)
  line L330 (-83.3931, -163.0784) -> (-85.8179, -163.0672)
  line L331 (-85.8179, -163.0672) -> (-87.0207, -160.9617)
  line L332 (-87.0207, -160.9617) -> (-85.7986, -158.8673)
  line L333 (-83.3738, 9.5783) -> (-82.171, 11.6839)
  line L334 (-85.7986, 9.5672) -> (-83.3738, 9.5783)
  line L335 (-87.0207, 11.6616) -> (-85.7986, 9.5672)
  line L336 (-85.8179, 13.7671) -> (-87.0207, 11.6616)
  line L337 (-83.3931, 13.7783) -> (-85.8179, 13.7671)
  line L338 (-82.171, 11.6839) -> (-83.3931, 13.7783)
  circle A2 centre (-84.5959, 11.6727) radius 1.1
  circle A3 centre (8.3275, 11.6727) radius 1.1
  line L339 (9.5302, 9.5672) -> (7.1054, 9.5783)
  line L340 (7.1054, 9.5783) -> (5.9026, 11.6839)
  line L341 (5.9026, 11.6839) -> (7.1247, 13.7783)
  line L342 (7.1247, 13.7783) -> (9.5496, 13.7671)
  line L343 (9.5496, 13.7671) -> (10.7523, 11.6616)
  line L344 (10.7523, 11.6616) -> (9.5302, 9.5672)
  point P0 (8.3275, -160.9728)
  dimension "d75" = 2.2
  dimension "d76" = 2.1
  constraint midpoint L312 L316.start
  constraint perpendicular L312 L316
  constraint perpendicular L32 L318
  constraint midpoint L313 L319.start
  constraint perpendicular L125 L319
  constraint perpendicular L313 L320
  constraint coincident P0 A0.centre
  constraint symmetric L318 A0 A1
  constraint symmetric L318 L321.start L328.end
  constraint symmetric L318 L321.end L329.end
  constraint symmetric L318 L322.end L330.end
  constraint symmetric L318 L323.end L331.end
  constraint symmetric L318 L324.end L327.start
  constraint symmetric L318 L325.end L327.end
  constraint symmetric L319 A0 A3
  constraint symmetric L319 L321.start L340.end
  constraint symmetric L319 L321.end L341.end
  constraint symmetric L319 L322.end L342.end
  constraint symmetric L319 L323.end L343.end
  constraint symmetric L319 L324.end L339.start
  constraint symmetric L319 L325.end L339.end
  constraint symmetric L319 A1 A2
  constraint symmetric L319 L327.start L334.start
  constraint symmetric L319 L327.end L333.start
  constraint symmetric L319 L328.end L333.end
  constraint symmetric L319 L329.end L337.start
  constraint symmetric L319 L330.end L336.start
  constraint symmetric L319 L331.end L335.start
  measures "d75" diameter of A0
  measures "d76" distance of P0 L326
extrude "Extrude25" cut sketch "Sketch9" against normal blind 90 contours A0 | A2 | A3 bodies 3
extrude "Extrude26" cut sketch "Sketch9" against normal blind 112 contours A1 bodies 3
extrude "Extrude27" cut sketch "Sketch9" against normal blind 70 from surface at -31 contours L321 L322 L323 L324 L325 L326 | L327 L328 L329 L330 L331 L332 bodies 3
extrude "Extrude28" cut sketch "Sketch9" against normal blind 10 from surface at -16 contours L333 L334 L335 L336 L337 L338 | L339 L340 L341 L342 L343 L344 bodies 3
sketch "Sketch10" plane through (0, 0, 1) normal (0, 0, 1) x (-1, 0, 0)
  line L0 (-82.4343, 9.2999) -> (-82.4343, -158.6)
  line L1 (-82.4343, -158.6) -> (6.1659, -158.6)
  line L2 (6.1659, -158.6) -> (6.1659, 9.2999)
  line L3 (6.1659, 9.2999) -> (-82.4343, 9.2999)
  circle A0 centre (-38.2354, -57.6876) radius 2
  circle A1 centre (-19.2847, -38.1233) radius 2
  circle A2 centre (-79.3226, -37.6472) radius 2
  circle A3 centre (-40.5598, 4.3284) radius 3.5
  circle A4 centre (-38.3065, -76.9092) radius 2
  circle A5 centre (-46.6015, -123.9891) radius 10
  circle A6 centre (-0.5822, -104.894) radius 5.0845
  circle A7 centre (-66.0181, -98.8044) radius 3
  circle A8 centre (1.6511, -57.8431) radius 3
  dimension "d87" = 4
  dimension "d88" = 4
  dimension "d89" = 4
  dimension "d90" = 7
  dimension "d91" = 4
  dimension "d92" = 20
  dimension "d93" = 6
  dimension "d94" = 6
  measures "d87" diameter of A0
  measures "d88" diameter of A1
  measures "d89" diameter of A2
  measures "d90" diameter of A3
  measures "d91" diameter of A4
  measures "d92" diameter of A5
  measures "d93" diameter of A7
  measures "d94" diameter of A8
extrude "Extrude29" add sketch "Sketch10" along normal blind 13.4 contours A0 | A1 | A2 | A3 | A4 | A5 | A6 | A7 | A8 bodies 3
named bodies: "plate"
